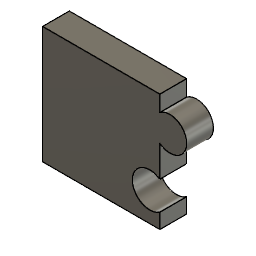
Test (Autodesk Fusion 360 archive; units mm, degrees)
design "Left"
Autodesk Fusion 360 part; units mm, degrees
sketch "Platform" plane through (0, 0, 0) normal (0, 1, 0) x (1, 0, 0)
  line L0 (35, -68) -> (35, -60)
  line L1 (0, -76) -> (0, -68)
  line L2 (0, -68) -> (35, -68)
  line L3 (35, -60) -> (0, -60)
  line L4 (35, -76) -> (0, -76)
  line L5 (0, -60) -> (0, -68)
  line L6 (35, -68) -> (35, -76)
  line L7 (0, -68) -> (35, -68)
  dimension "d1" = 8
  dimension "d2" = 35
  dimension "d3" = 60
  dimension "d4" = 8
  constraint horizontal L2
  constraint vertical L6
  constraint horizontal L4
  constraint vertical L1
  constraint coincident origin L1
  constraint horizontal L7
  constraint vertical L0
  constraint horizontal L3
  constraint vertical L5
  constraint equal L4 L7
  constraint coincident origin L5
  constraint collinear L2 L7
  measures "d1" distance of L2 L4
  measures "d2" distance of L1 L6
  measures "d3" distance of origin L3
  measures "d4" distance of L3 L7
extrude "Extrude1" add sketch "Platform" along normal mid plane 35 contours L1 L2 L4 L6 L7
sketch "Puzzle" plane through (0, 0, 68) normal (0, 0, -1) x (-1, 0, 0)
  line L0 (0, -17.5) -> (0, 17.5)
  line L1 (0, 17.5) -> (-35, 17.5)
  line L2 (-35, 17.5) -> (-35, -17.5)
  line L3 (-35, -17.5) -> (0, -17.5)
  circle A0 centre (-3, 8.75) radius 5.2
  line L4 (0, -17.5) -> (-35, 0) construction
  line L5 (-17.5, -17.5) -> (-17.5, 0) construction
  line L6 (0, -17.5) -> (0, 17.5)
  circle A1 centre (3, 8.75) radius 5 construction
  line L7 (-32, -13.95) -> (-32, -3.55) construction
  circle A2 centre (-32, -8.75) radius 5.2
  circle A3 centre (-32, 8.75) radius 5.2 construction
  circle A4 centre (-32, -8.75) radius 5 construction
  line L8 (0, 0) -> (-35, 0) construction
  line L9 (0, 0) -> (-35, -17.5) construction
  circle A5 centre (-38, 8.75) radius 5
  line L10 (0, 17.5) -> (-35, 17.5)
  circle A6 centre (3, -8.75) radius 5
  line L11 (3, -13.75) -> (3, -3.75) construction
  line L12 (-35, -17.5) -> (0, -17.5)
  line L13 (-35, 17.5) -> (-35, -17.5)
  point P0 (-17.5, -8.75)
  dimension "d11" = 10
  dimension "d12" = 3
  dimension "d13" = 3
  dimension "d14" = 0.2
  constraint coincident L11.start A6
  constraint coincident L11.end A6
  constraint vertical L11
  constraint coincident A6.centre L11
  constraint coincident L8.start L9.start
  constraint coincident L4.end L13
  constraint horizontal L8
  constraint coincident L0.start L3.end
  constraint coincident L2.end L3.start
  constraint midpoint P0 L4
  constraint horizontal P0 A6.centre
  constraint midpoint L5.start L12
  constraint midpoint L5.end L8
  constraint coincident L7.start A2
  constraint coincident L7.end A2
  constraint vertical L7
  constraint coincident A2.centre L7
  constraint horizontal A2.centre P0
  constraint symmetric A2 A3 L8
  constraint symmetric A0 L5 A3
  constraint symmetric A1 L8 A6
  constraint symmetric L5 A1 A5
  constraint equal A4 A6
  constraint coincident A2.centre A4.centre
  constraint coincident L0.end L1.start
  constraint coincident L1.end L2.start
  constraint coincident L9.start L8
  measures "d11" diameter of A6
  measures "d12" distance of L6 L11
  measures "d13" distance of L7 L13
  measures "d14" distance of A2 A4
sketch "Adapter" plane through (0, 0, 68) normal (0, 0, -1) x (-1, 0, 0)
  line L0 (-35, 17.5) -> (-35, -17.5)
  line L1 (-35, -17.5) -> (0, -17.5)
  line L2 (0, -17.5) -> (0, 17.5)
  line L3 (0, 17.5) -> (-35, 17.5)
  circle A0 centre (-17.5, -9) radius 3
  circle A1 centre (-17.5, 9) radius 3
  line L4 (0, -6) -> (-35, -6) construction
  circle A2 centre (-17.5, 9) radius 3.2
  line L5 (0, 0) -> (-35, 0) construction
  circle A3 centre (-17.5, -9) radius 3.2
  line L6 (-35, -17.5) -> (0, 0) construction
  line L7 (0, -17.5) -> (-35, 0) construction
  line L8 (-17.5, -8.75) -> (-17.5, 0) construction
  point P0 (-17.5, 0)
  dimension "d26" = 6
  dimension "d27" = 0.2
  dimension "d28" = 6
  constraint concentric A0 A3
  constraint coincident A1.centre A2.centre
  constraint vertical A0.centre P0
  constraint symmetric A0 A1 L5
  constraint symmetric A2 L5 A3
  constraint horizontal L4
  constraint tangent A0 L4
  constraint coincident L6.end L5
  constraint coincident P0 L5
  constraint coincident L0.end L1.start
  constraint coincident L5.start L6.end
  constraint coincident L1.end L2.start
  constraint midpoint L6 L8.start
  constraint midpoint L5 P0
  constraint coincident P0 L8
  constraint coincident L0 L5.end
  constraint coincident L0 L4.end
  constraint coincident L2 L4.start
  measures "d26" diameter of A0
  measures "d27" distance of A0 A3
  measures "d28" distance of L4 L5
extrude "Extrude6" cut sketch "Adapter" against normal blind 6 contours A0 | A1 | A2 | A3
chamfer "Chamfer1" distance 1.2 angle 45 2 edges at (20.4834, 10.1572, 74) (20.4834, -7.8428, 74)
extrude "PuzzleHoleLeft" [suppressed]
extrude "PuzzleHoleRight" cut sketch "Puzzle" against normal up to surface (8 mm away) contours L2 A2 L13 picked at (-32.7067, -7.5959)
extrude "PuzzleStumpLeft" [suppressed]
extrude "PuzzleStumpRight" add sketch "Puzzle" against normal blind 8 contours L2 A5 L13 picked at (-41.8863, 9.4989)
equation "d1 = PlatformHeight"
equation "d2 = LetterWidth"
equation "d3 = AdapterOffset"
equation "d4 = AdapterHeight"
equation "AdapterOffset = 60 mm"
equation "AdapterHeight = 8 mm"
equation "PlatformHeight = 8 mm"
equation "LetterWidth = 35 mm"
equation "d9 = LetterWidth"
equation "d11 = PuzzleRadius"
equation "d12 = PuzzleOffset"
equation "d13 = PuzzleOffset"
equation "d14 = Gap"
equation "PuzzleOffset = 3 mm"
equation "PuzzleRadius = 10 mm"
equation "Gap = 0.2 mm"
equation "d26 = AdapterHoleRadius"
equation "d27 = Gap"
equation "d28 = AdapterHoleSpread"
equation "AdapterHoleSpread = 6 mm"
equation "AdapterHoleRadius = 6 mm"
equation "AdapterHoleDepth = 6 mm"
equation "AdapterHoleBevel = 1.2 mm"
equation "d33 = -AdapterHoleDepth"
equation "d35 = AdapterHoleBevel"
equation "d45 = -PlatformHeight"
named bodies: "Platform"

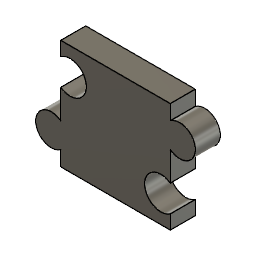
design "Platform"
part number: Center
Autodesk Fusion 360 part; units mm, degrees
sketch "Platform" plane through (0, 0, 0) normal (0, 1, 0) x (1, 0, 0)
  line L0 (35, -68) -> (35, -60)
  line L1 (0, -76) -> (0, -68)
  line L2 (0, -68) -> (35, -68)
  line L3 (35, -60) -> (0, -60)
  line L4 (35, -76) -> (0, -76)
  line L5 (0, -60) -> (0, -68)
  line L6 (35, -68) -> (35, -76)
  line L7 (0, -68) -> (35, -68)
  dimension "d1" = 8
  dimension "d2" = 35
  dimension "d3" = 60
  dimension "d4" = 8
  constraint horizontal L2
  constraint vertical L6
  constraint horizontal L4
  constraint vertical L1
  constraint coincident origin L1
  constraint horizontal L7
  constraint vertical L0
  constraint horizontal L3
  constraint vertical L5
  constraint equal L4 L7
  constraint coincident origin L5
  constraint collinear L2 L7
  measures "d1" distance of L2 L4
  measures "d2" distance of L1 L6
  measures "d3" distance of origin L3
  measures "d4" distance of L3 L7
extrude "Extrude1" add sketch "Platform" along normal mid plane 35 contours L1 L2 L4 L6 L7
sketch "Puzzle" plane through (0, 0, 68) normal (0, 0, -1) x (-1, 0, 0)
  line L0 (0, -17.5) -> (0, 17.5)
  line L1 (0, 17.5) -> (-35, 17.5)
  line L2 (-35, 17.5) -> (-35, -17.5)
  line L3 (-35, -17.5) -> (0, -17.5)
  circle A0 centre (-3, 8.75) radius 5.2
  line L4 (0, -17.5) -> (-35, 0) construction
  line L5 (-17.5, -17.5) -> (-17.5, 0) construction
  line L6 (0, -17.5) -> (0, 17.5)
  circle A1 centre (3, 8.75) radius 5 construction
  line L7 (-32, -13.95) -> (-32, -3.55) construction
  circle A2 centre (-32, -8.75) radius 5.2
  circle A3 centre (-32, 8.75) radius 5.2 construction
  circle A4 centre (-32, -8.75) radius 5 construction
  line L8 (0, 0) -> (-35, 0) construction
  line L9 (0, 0) -> (-35, -17.5) construction
  circle A5 centre (-38, 8.75) radius 5
  line L10 (0, 17.5) -> (-35, 17.5)
  circle A6 centre (3, -8.75) radius 5
  line L11 (3, -13.75) -> (3, -3.75) construction
  line L12 (-35, -17.5) -> (0, -17.5)
  line L13 (-35, 17.5) -> (-35, -17.5)
  point P0 (-17.5, -8.75)
  dimension "d11" = 10
  dimension "d12" = 3
  dimension "d13" = 3
  dimension "d14" = 0.2
  constraint coincident L11.start A6
  constraint coincident L11.end A6
  constraint vertical L11
  constraint coincident A6.centre L11
  constraint coincident L8.start L9.start
  constraint coincident L4.end L13
  constraint horizontal L8
  constraint coincident L0.start L3.end
  constraint coincident L2.end L3.start
  constraint midpoint P0 L4
  constraint horizontal P0 A6.centre
  constraint midpoint L5.start L12
  constraint midpoint L5.end L8
  constraint coincident L7.start A2
  constraint coincident L7.end A2
  constraint vertical L7
  constraint coincident A2.centre L7
  constraint horizontal A2.centre P0
  constraint symmetric A2 A3 L8
  constraint symmetric A0 L5 A3
  constraint symmetric A1 L8 A6
  constraint symmetric L5 A1 A5
  constraint equal A4 A6
  constraint coincident A2.centre A4.centre
  constraint coincident L0.end L1.start
  constraint coincident L1.end L2.start
  constraint coincident L9.start L8
  measures "d11" diameter of A6
  measures "d12" distance of L6 L11
  measures "d13" distance of L7 L13
  measures "d14" distance of A2 A4
sketch "Adapter" plane through (0, 0, 68) normal (0, 0, -1) x (-1, 0, 0)
  line L0 (-35, 17.5) -> (-35, -17.5)
  line L1 (-35, -17.5) -> (0, -17.5)
  line L2 (0, -17.5) -> (0, 17.5)
  line L3 (0, 17.5) -> (-35, 17.5)
  circle A0 centre (-17.5, -9) radius 3
  circle A1 centre (-17.5, 9) radius 3
  line L4 (0, -6) -> (-35, -6) construction
  circle A2 centre (-17.5, 9) radius 3.2
  line L5 (0, 0) -> (-35, 0) construction
  circle A3 centre (-17.5, -9) radius 3.2
  line L6 (-35, -17.5) -> (0, 0) construction
  line L7 (0, -17.5) -> (-35, 0) construction
  line L8 (-17.5, -8.75) -> (-17.5, 0) construction
  point P0 (-17.5, 0)
  dimension "d26" = 6
  dimension "d27" = 0.2
  dimension "d28" = 6
  constraint concentric A0 A3
  constraint coincident A1.centre A2.centre
  constraint vertical A0.centre P0
  constraint symmetric A0 A1 L5
  constraint symmetric A2 L5 A3
  constraint horizontal L4
  constraint tangent A0 L4
  constraint coincident L6.end L5
  constraint coincident P0 L5
  constraint coincident L0.end L1.start
  constraint coincident L5.start L6.end
  constraint coincident L1.end L2.start
  constraint midpoint L6 L8.start
  constraint midpoint L5 P0
  constraint coincident P0 L8
  constraint coincident L0 L5.end
  constraint coincident L0 L4.end
  constraint coincident L2 L4.start
  measures "d26" diameter of A0
  measures "d27" distance of A0 A3
  measures "d28" distance of L4 L5
extrude "Extrude6" cut sketch "Adapter" against normal blind 6 contours A0 | A1 | A2 | A3
chamfer "Chamfer1" distance 1.2 angle 45 2 edges at (20.4834, 10.1572, 74) (20.4834, -7.8428, 74)
extrude "PuzzleHoleLeft" cut sketch "Puzzle" against normal up to surface (8 mm away) contours L0 A0 L6 picked at (-2.715, 8.4983)
extrude "PuzzleHoleRight" cut sketch "Puzzle" against normal up to surface (8 mm away) contours L2 A2 L13 picked at (-32.7067, -7.5959)
extrude "PuzzleStumpLeft" add sketch "Puzzle" against normal up to surface (8 mm away) contours L0 L6 A6 picked at (2.5946, -9.2349)
extrude "PuzzleStumpRight" add sketch "Puzzle" against normal blind 8 contours L2 A5 L13 picked at (-41.8863, 9.4989)
equation "d1 = PlatformHeight"
equation "d2 = LetterWidth"
equation "d3 = AdapterOffset"
equation "d4 = AdapterHeight"
equation "AdapterOffset = 60 mm"
equation "AdapterHeight = 8 mm"
equation "PlatformHeight = 8 mm"
equation "LetterWidth = 35 mm"
equation "d9 = LetterWidth"
equation "d11 = PuzzleRadius"
equation "d12 = PuzzleOffset"
equation "d13 = PuzzleOffset"
equation "d14 = Gap"
equation "PuzzleOffset = 3 mm"
equation "PuzzleRadius = 10 mm"
equation "Gap = 0.2 mm"
equation "d26 = AdapterHoleRadius"
equation "d27 = Gap"
equation "d28 = AdapterHoleSpread"
equation "AdapterHoleSpread = 6 mm"
equation "AdapterHoleRadius = 6 mm"
equation "AdapterHoleDepth = 6 mm"
equation "AdapterHoleBevel = 1.2 mm"
equation "d33 = -AdapterHoleDepth"
equation "d35 = AdapterHoleBevel"
equation "d45 = -PlatformHeight"
named bodies: "Platform"

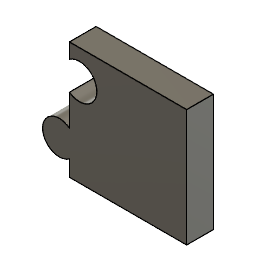
design "Right"
Autodesk Fusion 360 part; units mm, degrees
sketch "Platform" plane through (0, 0, 0) normal (0, 1, 0) x (1, 0, 0)
  line L0 (35, -68) -> (35, -60)
  line L1 (0, -76) -> (0, -68)
  line L2 (0, -68) -> (35, -68)
  line L3 (35, -60) -> (0, -60)
  line L4 (35, -76) -> (0, -76)
  line L5 (0, -60) -> (0, -68)
  line L6 (35, -68) -> (35, -76)
  line L7 (0, -68) -> (35, -68)
  dimension "d1" = 8
  dimension "d2" = 35
  dimension "d3" = 60
  dimension "d4" = 8
  constraint horizontal L2
  constraint vertical L6
  constraint horizontal L4
  constraint vertical L1
  constraint coincident origin L1
  constraint horizontal L7
  constraint vertical L0
  constraint horizontal L3
  constraint vertical L5
  constraint equal L4 L7
  constraint coincident origin L5
  constraint collinear L2 L7
  measures "d1" distance of L2 L4
  measures "d2" distance of L1 L6
  measures "d3" distance of origin L3
  measures "d4" distance of L3 L7
extrude "Extrude1" add sketch "Platform" along normal mid plane 35 contours L1 L2 L4 L6 L7
sketch "Puzzle" plane through (0, 0, 68) normal (0, 0, -1) x (-1, 0, 0)
  line L0 (0, -17.5) -> (0, 17.5)
  line L1 (0, 17.5) -> (-35, 17.5)
  line L2 (-35, 17.5) -> (-35, -17.5)
  line L3 (-35, -17.5) -> (0, -17.5)
  circle A0 centre (-3, 8.75) radius 5.2
  line L4 (0, -17.5) -> (-35, 0) construction
  line L5 (-17.5, -17.5) -> (-17.5, 0) construction
  line L6 (0, -17.5) -> (0, 17.5)
  circle A1 centre (3, 8.75) radius 5 construction
  line L7 (-32, -13.95) -> (-32, -3.55) construction
  circle A2 centre (-32, -8.75) radius 5.2
  circle A3 centre (-32, 8.75) radius 5.2 construction
  circle A4 centre (-32, -8.75) radius 5 construction
  line L8 (0, 0) -> (-35, 0) construction
  line L9 (0, 0) -> (-35, -17.5) construction
  circle A5 centre (-38, 8.75) radius 5
  line L10 (0, 17.5) -> (-35, 17.5)
  circle A6 centre (3, -8.75) radius 5
  line L11 (3, -13.75) -> (3, -3.75) construction
  line L12 (-35, -17.5) -> (0, -17.5)
  line L13 (-35, 17.5) -> (-35, -17.5)
  point P0 (-17.5, -8.75)
  dimension "d11" = 10
  dimension "d12" = 3
  dimension "d13" = 3
  dimension "d14" = 0.2
  constraint coincident L11.start A6
  constraint coincident L11.end A6
  constraint vertical L11
  constraint coincident A6.centre L11
  constraint coincident L8.start L9.start
  constraint coincident L4.end L13
  constraint horizontal L8
  constraint coincident L0.start L3.end
  constraint coincident L2.end L3.start
  constraint midpoint P0 L4
  constraint horizontal P0 A6.centre
  constraint midpoint L5.start L12
  constraint midpoint L5.end L8
  constraint coincident L7.start A2
  constraint coincident L7.end A2
  constraint vertical L7
  constraint coincident A2.centre L7
  constraint horizontal A2.centre P0
  constraint symmetric A2 A3 L8
  constraint symmetric A0 L5 A3
  constraint symmetric A1 L8 A6
  constraint symmetric L5 A1 A5
  constraint equal A4 A6
  constraint coincident A2.centre A4.centre
  constraint coincident L0.end L1.start
  constraint coincident L1.end L2.start
  constraint coincident L9.start L8
  measures "d11" diameter of A6
  measures "d12" distance of L6 L11
  measures "d13" distance of L7 L13
  measures "d14" distance of A2 A4
sketch "Adapter" plane through (0, 0, 68) normal (0, 0, -1) x (-1, 0, 0)
  line L0 (-35, 17.5) -> (-35, -17.5)
  line L1 (-35, -17.5) -> (0, -17.5)
  line L2 (0, -17.5) -> (0, 17.5)
  line L3 (0, 17.5) -> (-35, 17.5)
  circle A0 centre (-17.5, -9) radius 3
  circle A1 centre (-17.5, 9) radius 3
  line L4 (0, -6) -> (-35, -6) construction
  circle A2 centre (-17.5, 9) radius 3.2
  line L5 (0, 0) -> (-35, 0) construction
  circle A3 centre (-17.5, -9) radius 3.2
  line L6 (-35, -17.5) -> (0, 0) construction
  line L7 (0, -17.5) -> (-35, 0) construction
  line L8 (-17.5, -8.75) -> (-17.5, 0) construction
  point P0 (-17.5, 0)
  dimension "d26" = 6
  dimension "d27" = 0.2
  dimension "d28" = 6
  constraint concentric A0 A3
  constraint coincident A1.centre A2.centre
  constraint vertical A0.centre P0
  constraint symmetric A0 A1 L5
  constraint symmetric A2 L5 A3
  constraint horizontal L4
  constraint tangent A0 L4
  constraint coincident L6.end L5
  constraint coincident P0 L5
  constraint coincident L0.end L1.start
  constraint coincident L5.start L6.end
  constraint coincident L1.end L2.start
  constraint midpoint L6 L8.start
  constraint midpoint L5 P0
  constraint coincident P0 L8
  constraint coincident L0 L5.end
  constraint coincident L0 L4.end
  constraint coincident L2 L4.start
  measures "d26" diameter of A0
  measures "d27" distance of A0 A3
  measures "d28" distance of L4 L5
extrude "Extrude6" cut sketch "Adapter" against normal blind 6 contours A0 | A1 | A2 | A3
chamfer "Chamfer1" distance 1.2 angle 45 2 edges at (20.4834, 10.1572, 74) (20.4834, -7.8428, 74)
extrude "PuzzleHoleLeft" cut sketch "Puzzle" against normal up to surface (8 mm away) contours L0 A0 L6 picked at (-2.715, 8.4983)
extrude "PuzzleHoleRight" [suppressed]
extrude "PuzzleStumpLeft" add sketch "Puzzle" against normal up to surface (8 mm away) contours L0 L6 A6 picked at (2.5946, -9.2349)
extrude "PuzzleStumpRight" [suppressed]
equation "d1 = PlatformHeight"
equation "d2 = LetterWidth"
equation "d3 = AdapterOffset"
equation "d4 = AdapterHeight"
equation "AdapterOffset = 60 mm"
equation "AdapterHeight = 8 mm"
equation "PlatformHeight = 8 mm"
equation "LetterWidth = 35 mm"
equation "d9 = LetterWidth"
equation "d11 = PuzzleRadius"
equation "d12 = PuzzleOffset"
equation "d13 = PuzzleOffset"
equation "d14 = Gap"
equation "PuzzleOffset = 3 mm"
equation "PuzzleRadius = 10 mm"
equation "Gap = 0.2 mm"
equation "d26 = AdapterHoleRadius"
equation "d27 = Gap"
equation "d28 = AdapterHoleSpread"
equation "AdapterHoleSpread = 6 mm"
equation "AdapterHoleRadius = 6 mm"
equation "AdapterHoleDepth = 6 mm"
equation "AdapterHoleBevel = 1.2 mm"
equation "d33 = -AdapterHoleDepth"
equation "d35 = AdapterHoleBevel"
equation "d45 = -PlatformHeight"
named bodies: "Platform"
